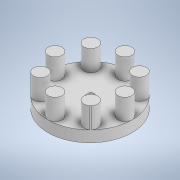
# Autodesk Inventor part: wheel
Saved by Autodesk Inventor 2022 (Build 260153000, 153)
## iProperties
Created: 2021-04-16
Part Number: wheel
Material: Generic
Document SubType Name: Modeling
Designer: kevin
Density: 1 g/cm^3
Appearance: Default
Author: kevin
Autodesk Inventor part; units mm, degrees
ref_plane "YZ Plane" through (0, 0, 0) normal (1, 0, 0) x (0, 1, 0)
ref_plane "XZ Plane" through (0, 0, 0) normal (0, 1, 0) x (-1, 0, 0)
ref_plane "XY Plane" through (0, 0, 0) normal (0, 0, 1) x (1, 0, 0)
sketch "Sketch1" plane through (0, 0, 0) normal (0, 1, 0) x (-1, 0, 0)
  circle A0 centre (0, 0) radius 38.1
  circle A1 centre (0, 0) radius 3.5719
  line L0 (2.6623, 2.3813) -> (2.6623, -2.3812)
  line L1 (2.6623, 0) -> (-3.5719, 0) construction
  dimension "d0" = 7.1437
  dimension "d1" = 76.2
  dimension "d2" = 4.7625
  dimension "d3" = 6.2342
  constraints: 4 end point, 3 point on circle, 2 centre point, 2 coincident, 1 horizontal, 1 midpoint, 1 vertical
  measures "d0" diameter of A1
  measures "d1" diameter of A0
  measures "d2" distance of L0.start L0.end
  measures "d3" distance of L1.start L1.end
extrude "main shape" add sketch "Sketch1" along normal blind 10.16 contours A0 | A1 L0 picked at (2.8274, 0.5567)
sketch "Sketch2" plane through (0, 10.16, 0) normal (0, 1, 0) x (1, 0, 0)
  circle A0 centre (0, 0) radius 38.1 projected
  arc A1 (22.0902, 31.0424) -> (31.0426, 22.0899) centre (26.9409, 26.9406) ccw construction
  line L0 (0, 38.1) -> (26.9409, 26.9406) construction
  line L1 (38.1, 0) -> (26.9409, 26.9406) construction
  line L2 (0, 38.1) -> (0, 0) construction
  line L3 (38.1, 0) -> (-38.1, 0) construction
  arc A2 (-6.3279, 37.5708) -> (6.3279, 37.5708) centre (0, 38.1) ccw construction
  arc A3 (-37.5708, -6.3279) -> (-37.5708, 6.3279) centre (-38.1, 0) ccw construction
  arc A4 (-31.0426, 22.0899) -> (-22.0902, 31.0424) centre (-26.9409, 26.9406) ccw construction
  arc A5 (6.3279, -37.5708) -> (-6.3279, -37.5708) centre (0, -38.1) ccw construction
  arc A6 (37.5708, 6.3279) -> (37.5708, -6.3279) centre (38.1, 0) ccw construction
  arc A7 (31.0426, -22.0899) -> (22.0902, -31.0424) centre (26.9409, -26.9406) ccw construction
  arc A8 (-22.0902, -31.0424) -> (-31.0426, -22.0899) centre (-26.9409, -26.9406) ccw construction
  arc A9 (-37.5708, -6.3279) -> (-37.5708, 6.3279) centre (-38.1, 0) ccw construction
  circle A10 centre (-31.75, 0) radius 6.35
  circle A11 centre (-22.0902, 22.8389) radius 6.3525
  circle A12 centre (0, 31.75) radius 6.35
  circle A13 centre (22.449, 22.4488) radius 6.3525
  circle A14 centre (31.75, 0) radius 6.35
  circle A15 centre (22.8391, -22.0899) radius 6.3525
  circle A16 centre (0, -31.75) radius 6.35
  circle A17 centre (-22.0902, -22.8389) radius 6.3525
  point P0 (-31.0426, -22.0899)
  point P1 (-26.9409, -26.9406)
  point P2 (-26.0281, -27.8235)
  point P3 (26.9409, -26.9406)
  point P4 (27.8239, -26.0277)
  point P5 (-26.9409, 26.9406)
  point P6 (-26.0281, 27.8235)
  dimension "d6" = 26.9409
  dimension "d7" = 26.9407
  constraints: 26 point on circle, 20 symmetric about line, 10 centre point, 8 end point, 2 horizontal alignment, 2 vertical alignment, 1 horizontal, 32 other
  measures "d6" horizontal distance of L0.start L0.end
  measures "d7" vertical distance of L1.start L0.end
extrude "pegs" add sketch "Sketch2" along normal blind 19.05 contours A13 | A12 | A10 | A16 | A14 | A0 A15 | A11 A0 | A0 A17 picked at (21.4863, -20.4795) picked at (-20.8028, 21.1724) picked at (-20.8028, -21.1724)
body "Solid1"
